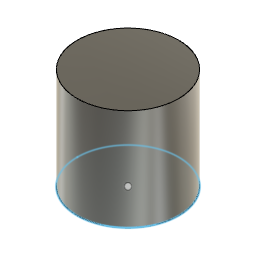
Small Pilon (Autodesk Fusion 360 design; units mm, degrees)
Autodesk Fusion 360 part; units mm, degrees
sketch "sketch 262" plane through (0, 0, 15) normal (0, 0, 1) x (-1, 0, 0)
  circle A0 centre (-87.5, -105) radius 2.5
  circle A1 centre (-87.5, -105) radius 2.5
extrude "Extrude1" add sketch "sketch 262" along normal blind 5
